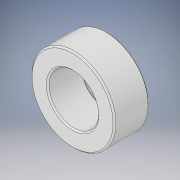
# Autodesk Inventor part: 3d printed nut
Saved by Autodesk Inventor 2019 (Build 230136000, 136)
## iProperties
Created: 2019-03-20
Part Number: 3d printed nut
Material: ABS Plastic
Document SubType Name: Modeling
Designer: pctech
Density: 1.06 g/cm^3
Appearance: Smooth - White
Author: pctech
Autodesk Inventor part; units mm, degrees
ref_plane "YZ Plane" through (0, 0, 0) normal (1, 0, 0) x (0, 1, 0)
ref_plane "XZ Plane" through (0, 0, 0) normal (0, 1, 0) x (-1, 0, 0)
ref_plane "XY Plane" through (0, 0, 0) normal (0, 0, 1) x (1, 0, 0)
sketch "Sketch1" plane through (0, 0, 0) normal (0, 0, 1) x (1, 0, 0)
  circle A0 centre (0, 0) radius 11.43
  circle A1 centre (0, 0) radius 6.7469
  dimension "d0" = 22.86
  dimension "d1" = 13.4938
  constraints: 2 centre point, 2 coincident
  measures "d0" diameter of A0
  measures "d1" diameter of A1
extrude "Extrusion1" add sketch "Sketch1" along normal mid plane 9.525
chamfer "Chamfer1" distance 0.4 angle 45 4 edges at (-11.43, 0, 4.7625) (-11.43, 0, -4.7625) (-6.7469, 0, 4.7625) (-6.7469, 0, -4.7625)
sketch "Sketch2" plane through (0, 0, 0) normal (1, 0, 0) x (0, 1, 0)
  point P0 (0, 0)
body "Solid1"
